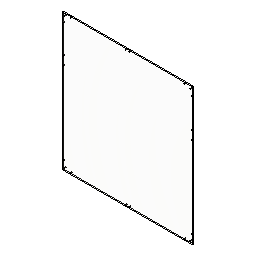
bottom250 v2 (Autodesk Fusion 360 design; units mm, degrees)
Autodesk Fusion 360 part; units mm, degrees
sketch "Sketch1" plane through (0, 0, 0) normal (0, 0, 1) x (1, 0, 0)
  line L0 (285.2, -298.2) -> (-285.2, -298.2)
  line L1 (-285.2, -298.2) -> (-285.2, 298.2)
  line L2 (-285.2, 298.2) -> (285.2, 298.2)
  line L3 (285.2, 298.2) -> (285.2, -298.2)
  line L4 (285.2, -298.2) -> (-285.2, 298.2) construction
  line L5 (-285.2, -298.2) -> (285.2, 298.2) construction
  circle A0 centre (-247.5, 294.2) radius 2
  circle A1 centre (-280.2, 260.5) radius 2
  circle A2 centre (-247.5, -293.2) radius 2
  circle A3 centre (-280.2, -260.5) radius 2
  circle A4 centre (247.5, 293.2) radius 2
  circle A5 centre (280.2, 260.5) radius 2
  circle A6 centre (247.5, -293.2) radius 2
  circle A7 centre (280.2, -260.5) radius 2
  line L6 (0, -298.2) -> (0, 298.2) construction
  circle A8 centre (8, 293.2) radius 2
  circle A9 centre (8, -293.2) radius 2
  circle A10 centre (-274.4128, -286.9211) radius 2
  circle A11 centre (274.4128, -286.9211) radius 2
  circle A12 centre (274.4128, 286.9211) radius 2
  circle A13 centre (-274.4128, 286.9211) radius 2
  circle A14 centre (-8, -293.2) radius 2
  circle A15 centre (-8, 293.2) radius 2
  line L7 (285.2, 114.4) -> (-285.2, 114.4) construction
  circle A16 centre (280.2, 95.6) radius 2
  circle A17 centre (280.2, 133.2) radius 2
  circle A18 centre (-280.2, 133.2) radius 2
  circle A19 centre (-280.2, 95.6) radius 2
  dimension "d1" = 570.4
  dimension "d2" = 596.4
  dimension "d4" = 4
  dimension "d5" = 4
  dimension "d6" = 4
  dimension "d7" = 37.7
  dimension "d8" = 4
  dimension "d9" = 4
  dimension "d13" = 4
  dimension "d14" = 4
  dimension "d17" = 4
  dimension "d18" = 4
  dimension "d23" = 4
  dimension "d24" = 4
  dimension "d25" = 5
  dimension "d26" = 5
  dimension "d30" = 5
  dimension "d31" = 5
  dimension "d32" = 4
  dimension "d33" = 15.607
  dimension "d34" = 5
  dimension "d35" = 5
  dimension "d36" = 37.7
  dimension "d37" = 37.7
  dimension "d38" = 37.7
  dimension "d39" = 37.7
  dimension "d40" = 4
  dimension "d41" = 15.607
  dimension "d42" = 5
  dimension "d43" = 37.7
  dimension "d44" = 5
  dimension "d45" = 37.7
  dimension "d46" = 4
  dimension "d47" = 15.607
  dimension "d48" = 4
  dimension "d49" = 15.607
  dimension "d50" = 37.7
  dimension "d51" = 5
  dimension "d52" = 4
  dimension "d53" = 8
  dimension "d54" = 8
  dimension "d55" = 5
  dimension "d56" = 8
  dimension "d57" = 4
  dimension "d58" = 8
  dimension "d59" = 5
  dimension "d60" = 412.6
  dimension "d61" = 4
  dimension "d62" = 4
  dimension "d63" = 18.8
  dimension "d64" = 18.8
  dimension "d65" = 5
  dimension "d66" = 5
  dimension "d67" = 4
  dimension "d68" = 4
  dimension "d69" = 18.8
  dimension "d70" = 18.8
  dimension "d71" = 5
  dimension "d72" = 5
  measures "d4" diameter of A0
  measures "d6" diameter of A1
  measures "d8" diameter of A2
  measures "d9" diameter of A3
  measures "d13" diameter of A4
  measures "d14" diameter of A5
  measures "d17" diameter of A6
  measures "d18" diameter of A7
  measures "d23" diameter of A8
  measures "d24" diameter of A9
  measures "d32" diameter of A10
  measures "d40" diameter of A11
  measures "d46" diameter of A12
  measures "d48" diameter of A13
  measures "d52" diameter of A14
  measures "d53" distance of L6
  measures "d54" distance of L6
  measures "d56" distance of L6
  measures "d57" diameter of A15
  measures "d58" distance of L6
  measures "d60" distance of L0 L7
  measures "d61" diameter of A16
  measures "d62" diameter of A17
  measures "d67" diameter of A18
  measures "d68" diameter of A19
extrude "Extrude1" add sketch "Sketch1" along normal blind 5 makes body 1
copy_body "Body->Comp1" bodies 1 removing the originals makes body 2 in component "Bottom"
component "Bottom" placed x (1, 0, 0) y (0, 1, 0) z (0, 0, 1) at (0, 0, 0)
equation "d1 = XRailLength + 220.4 mm"
equation "d2 = YRailLength + 246.4 mm"
equation "d60 = YRailLength + 62.6 mm"
equation "d63 = ( 37.6 / 2 ) * 1 mm"
equation "d64 = ( 37.6 / 2 ) * 1 mm"
equation "d69 = ( 37.6 / 2 ) * 1 mm"
equation "d70 = ( 37.6 / 2 ) * 1 mm"
equation "XRailLength = 350 mm"
equation "YRailLength = 350 mm"
named bodies: "Bottom"
